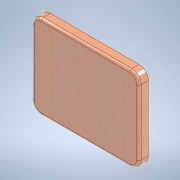
# Autodesk Inventor part: stand
Saved by Autodesk Inventor 2021.1 (Build 251245000, 245)
## iProperties
Created: 2020-08-27
Part Number: stand
Material: Wood (Oak)
Document SubType Name: Sheet Metal
Designer: Vamshi
Mass: 10226.5 g
Surface Area: 6311.38 cm^2
Volume: 13456 cm^3
Density: 0.76 g/cm^3
Sheet Metal Rule: Default
Appearance: White Oak - Natural Medium Gloss
Author: Vamshi
Autodesk Inventor part; units mm, degrees
ref_plane "YZ Plane" through (0, 0, 0) normal (1, 0, 0) x (0, 1, 0)
ref_plane "XZ Plane" through (0, 0, 0) normal (0, 1, 0) x (-1, 0, 0)
ref_plane "XY Plane" through (0, 0, 0) normal (0, 0, 1) x (1, 0, 0)
sketch "Sketch1" plane through (0, 0, 0) normal (0, 0, 1) x (1, 0, 0)
  line L0 (39.2805, 6.8884) -> (521.8805, 6.8884)
  line L1 (572.6805, -43.9116) -> (572.6805, -399.5116)
  line L2 (521.8805, -450.3116) -> (39.2805, -450.3116)
  line L3 (-11.5195, -399.5116) -> (-11.5195, -43.9116)
  arc A0 (-11.5195, -399.5116) -> (39.2805, -450.3116) centre (39.2805, -399.5116) ccw
  arc A1 (39.2805, 6.8884) -> (-11.5195, -43.9116) centre (39.2805, -43.9116) ccw
  arc A2 (572.6805, -43.9116) -> (521.8805, 6.8884) centre (521.8805, -43.9116) ccw
  arc A3 (521.8805, -450.3116) -> (572.6805, -399.5116) centre (521.8805, -399.5116) ccw
  circle A4 centre (471.0805, -145.5116) radius 22.86
  circle A5 centre (471.0805, -145.5116) radius 13.97
  line L4 (280.5805, -450.3116) -> (280.5805, 6.8884)
  line L5 (-11.5195, -221.7116) -> (572.6805, -221.7116)
  circle A6 centre (90.0805, -145.5116) radius 22.86
  circle A7 centre (90.0805, -145.5116) radius 13.97
  circle A8 centre (471.0805, -297.9116) radius 22.86
  circle A9 centre (471.0805, -297.9116) radius 13.97
  circle A10 centre (90.0805, -297.9116) radius 13.97
  circle A11 centre (90.0805, -297.9116) radius 22.86
  point P0 (0, 0)
  point P1 (572.6805, -450.3116)
  point P2 (572.6805, 6.8884)
  point P3 (-11.5195, -450.3116)
  dimension "d0" = 584.2
  dimension "d1" = 457.2
  dimension "d2" = 50.8
  dimension "d3" = 50.8
  dimension "d7" = 45.72
  dimension "d8" = 27.94
  dimension "d9" = 152.4
  dimension "d10" = 101.6
  constraints: 12 centre point, 12 end point, 8 point on circle, 8 tangent, 6 point on line, 6 symmetric about line, 4 coincident, 4 midpoint, 2 equal radius, 2 parallel, 1 horizontal, 1 perpendicular, 6 other
  measures "d0" distance of point (572.681, -450.312) point (-11.519, -450.312)
  measures "d1" distance of point (572.681, 6.888) point (572.681, -450.312)
  measures "d2" radius of A0
  measures "d3" radius of A1
  measures "d7" diameter of A4
  measures "d8" diameter of A5
  measures "d9" distance from line of L0 A4.centre
  measures "d10" distance from line of L1 A4.centre
extrude "Extrusion1" add sketch "Sketch1" along normal blind 50.8 contours L0 L4 L5 L3 A1 | L0 A2 L1 L5 L4 | L5 L1 A3 L2 L4 | L4 L2 A0 L3 L5 | A4 | A5 | A6 | A7 | A8 | A9 | A10 | A11
fillet "Fillet1" radius 12.7 8 edges at (3.3595, -7.9905, 50.8) (-11.5195, -221.7116, 50.8) (3.3595, -435.4326, 50.8) (280.5805, -450.3116, 50.8) (557.8015, -435.4326, 50.8) (572.6805, -221.7116, 50.8) (557.8015, -7.9905, 50.8) (280.5805, 6.8884, 50.8)
sketch "Sketch2" plane through (0, 0, 0) normal (0, 0, -1) x (-1, 0, 0)
  point P0 (0, 0)
equation "\"BendRadius\" = Thickness"
equation "\"BendReliefWidth\" = Thickness"
equation "\"BendReliefDepth\" = 0.5 * Thickness"
equation "\"CornerReliefSize\" = 4 * Thickness"
equation "\"MinimumRemnant\" = 2 * Thickness"
equation "\"TransitionRadius\" = BendRadius"
equation "\"JacobiRadiusSize\" = BendRadius"
equation "\"GapSize\" = Thickness"
equation "\"Thickness\" = 3.048"
body "Solid1"
